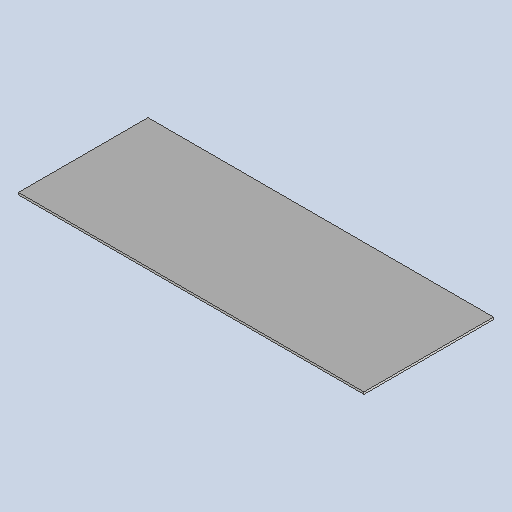
# Autodesk Inventor part: TRM 038 facr wall
Saved by Autodesk Inventor 2025 (Build 290162010, 162A)
## iProperties
Created: 2024-08-07
Part Number: TRM 038 facr wall
Material: AISI 304
Document SubType Name: Sheet Metal
Designer: user
Stock Number: ТРМ 012 спина основное
Mass: 2080.77 g
Surface Area: 1767.6 cm^2
Volume: 259.2 cm^3
Density: 8.02768 g/cm^3
Flat Pattern Width: 48 cm
Flat Pattern Length: 18 cm
Flat Pattern Area: 864 cm^2
Sheet Metal Rule: AISI304 2mm Die16
Sheet Metal Width: 480.000 mm
Sheet Metal Length: 180.000 mm
Sheet Metal Area: 86400.000 mm^2
Appearance: Default
Author: pokla
Autodesk Inventor part; units mm, degrees
ref_plane "YZ Plane" through (0, 0, 0) normal (1, 0, 0) x (0, 1, 0)
ref_plane "XZ Plane" through (0, 0, 0) normal (0, 1, 0) x (-1, 0, 0)
ref_plane "XY Plane" through (0, 0, 0) normal (0, 0, 1) x (1, 0, 0)
sketch "Sketch1" plane through (0, 0, 0) normal (0, 0, 1) x (1, 0, 0)
  line L0 (-240, -90) -> (240, -90)
  line L1 (240, -90) -> (240, 90)
  line L2 (240, 90) -> (-240, 90)
  line L3 (-240, 90) -> (-240, -90)
  line L4 (-240, -90) -> (240, 90) construction
  line L5 (240, -90) -> (-240, 90) construction
  point P0 (0, 0)
  dimension "d0" = 480
  dimension "d1" = 180
  measures "d0" distance of L2.end L1.end
  measures "d1" distance of L1.end L0.end
extrude "Plate1" add sketch "Sketch1" along normal blind 3
sketch "Sketch2" plane through (0, 0, 0) normal (0, 0, -1) x (-1, 0, 0)
  line L0 (-220, 70) -> (-20, 70) construction
  line L1 (-20, 70) -> (-20, 50) construction
  line L2 (-20, 50) -> (-220, 50) construction
  line L3 (-220, 50) -> (-220, 70) construction
  line L4 (-240, 90) -> (240, 90) projected
  line L5 (-240, -90) -> (-240, 90) projected
  point P0 (0, 0)
  point P1 (-220, 60)
  dimension "d6" = 200
  dimension "d7" = 20
  dimension "d8" = 20
  dimension "d9" = 20
  constraints: 1 midpoint, 2 other
  measures "d6" distance of L0.start L0.end
  measures "d7" distance of L0.end L1.end
  measures "d8" distance between parallel lines of L4 L0
  measures "d9" distance from line of L5 point (-220, 60)
mark "Mark1"
equation "\"d2\" = Thickness"
equation "\"BendReliefWidth\" = Thickness"
equation "\"BendReliefDepth\" = 0.5 * Thickness"
equation "\"CornerReliefSize\" = 4 * Thickness"
equation "\"MinimumRemnant\" = 2 * Thickness"
equation "\"TransitionRadius\" = BendRadius"
equation "\"JacobiRadiusSize\" = BendRadius"
equation "\"GapSize\" = Thickness"
equation "\"Thickness\" = 3"
equation "\"BendRadius\" = 2.75"
body "Solid1"
